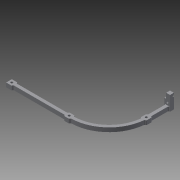
# Autodesk Inventor part: UndercarriageLeft
Saved by Autodesk Inventor 2014 SP1 (Build 180222100, 222)
## iProperties
Created: 2017-01-18
Part Number: UndercarriageLeft
Material: Generic
Document SubType Name: Modeling
Designer: danielsikar
Density: 1 g/cm^3
Appearance: Default
d38: 5.000 mm
d39: 200.000 mm
d40: 125.500 mm
d41: 11.000 mm
d42: 11.000 mm
d43: 11.000 mm
d44: 5.000 mm
d45: 6.000 mm
d46: 6.000 mm
d47: 150.000 mm
d48: 150.000 mm
d51: 6.000 mm
d52: 0.00 deg
d53: 4.300 mm
d54: 6.000 mm
d55: 0.00 deg
d56: 10.000 mm
d57: 0.00 deg
d58: 4.300 mm
d59: 5.000 mm
d60: 10.000 mm
d61: 0.00 deg
d62: 5.000 mm
d63: 10.000 mm
d64: 0.00 deg
d65: 4.300 mm
d66: 5.000 mm
d67: 10.000 mm
d68: 0.00 deg
d69: 11.000 mm
d70: 11.000 mm
d71: 6.000 mm
d72: 0.00 deg
d73: 4.300 mm
d74: 6.000 mm
d75: 0.00 deg
d76: 2.000 mm
d77: 2.000 mm
d80: 11.000 mm
d81: 11.000 mm
d82: 6.000 mm
d83: 0.00 deg
d84: 4.300 mm
d85: 6.000 mm
d86: 0.00 deg
d87: 2.000 mm
d88: 2.500 mm
d89: 0.00 deg
d98: 2.500 mm
d99: 0.00 deg
d100: 2.000 mm
d101: 2.000 mm
d102: 0.00 deg
Author: danielsikar
Autodesk Inventor part; units mm, degrees
ref_plane "YZ Plane" through (0, 0, 0) normal (1, 0, 0) x (0, 1, 0)
ref_plane "XZ Plane" through (0, 0, 0) normal (0, 1, 0) x (-1, 0, 0)
ref_plane "XY Plane" through (0, 0, 0) normal (0, 0, 1) x (1, 0, 0)
sketch "Sketch8" plane through (0, 0, 0) normal (0, 0, 1) x (1, 0, 0)
  line L0 (0, 0) -> (200, 0) construction
  line L1 (200, 0) -> (200, 125.5) construction
  line L2 (200, 125.5) -> (0, 125.5) construction
  line L3 (0, 125.5) -> (0, 0) construction
  line L4 (0, 0) -> (11, 0)
  line L5 (11, 11) -> (0, 11)
  line L6 (0, 11) -> (0, 0)
  line L7 (200, 125.5) -> (189, 125.5)
  line L8 (189, 125.5) -> (189, 120.5)
  line L9 (200, 120.5) -> (200, 125.5)
  line L10 (217.9822, 8.5) -> (217.9822, 2.5)
  line L11 (-10.7087, 2.5) -> (-10.7087, 8.5)
  line L12 (191.5, 137.3826) -> (197.5, 137.3826)
  line L13 (197.5, -11.2875) -> (191.5, -11.2875)
  line L14 (197.5, 2.5) -> (47.5, 2.5) construction
  line L15 (47.5, 2.5) -> (47.5, 152.5) construction
  line L16 (47.5, 152.5) -> (197.5, 152.5) construction
  line L17 (122.5, 152.5) -> (122.5, -14.6568) construction
  line L18 (47.5, 77.5) -> (239.0403, 77.5) construction
  circle A0 centre (122.5, 77.5) radius 69
  line L19 (-10.7087, 8.5) -> (0, 8.5)
  line L20 (217.9822, 2.5) -> (11, 2.5)
  line L21 (0, 2.5) -> (-10.7087, 2.5)
  line L22 (11, 0) -> (11, 2.5)
  line L23 (11, 8.5) -> (11, 11)
  line L24 (11, 8.5) -> (122.5, 8.5)
  line L25 (151.8939, 8.5) -> (217.9822, 8.5)
  line L26 (191.5, -11.2875) -> (191.5, 8.5)
  arc A1 (122.5, 2.5) -> (197.5, 77.5) centre (122.5, 77.5) ccw
  arc A2 (191.5, 106.8939) -> (93.1061, 8.5) centre (122.5, 77.5) ccw
  line L27 (189, 120.5) -> (191.5, 120.5)
  line L28 (197.5, 120.5) -> (200, 120.5)
  line L29 (191.5, 77.5) -> (191.5, 120.5)
  line L30 (191.5, 125.5) -> (191.5, 137.3826)
  line L31 (197.5, 152.5) -> (197.5, 125.5) construction
  line L32 (197.5, 120.5) -> (197.5, 2.5) construction
  line L33 (197.5, 137.3826) -> (197.5, 125.5)
  line L34 (197.5, 120.5) -> (197.5, 77.5)
  line L35 (197.5, 8.5) -> (197.5, -11.2875)
  point P0 (-10.7087, 5.5)
  point P1 (0, 5.5)
  point P2 (194.5, 137.3826)
  point P3 (194.5, 125.5)
  dimension "d39" = 200
  dimension "d40" = 125.5
  dimension "d41" = 11
  dimension "d42" = 11
  dimension "d43" = 11
  dimension "d44" = 5
  dimension "d45" = 6
  dimension "d46" = 6
  dimension "d47" = 150
  dimension "d48" = 150
  constraints: 72 end point, 28 parallel, 14 point on line, 13 perpendicular, 8 horizontal, 7 point on circle, 6 midpoint, 5 tangent, 3 centre point, 1 coincident, 1 horizontal alignment, 1 vertical alignment
  measures "d39" distance of L2.end L1.end
  measures "d40" distance of L1.end L0.end
  measures "d41" distance of L5.end L5.start
  measures "d42" distance of L5.start L4.end
  measures "d43" distance of L9.start L8.end
  measures "d44" distance of L8.end L7.end
  measures "d45" distance of L10.start L10.end
  measures "d46" distance of L13.start L13.end
  measures "d47" distance of L15.end L16.end
  measures "d48" distance of L14.end L15.end
extrude "Extrusion8" add sketch "Sketch8" along normal blind 6 contours L6 L5 L23 L24 A0 L29 L27 L8 L7 L9 L28 L34 A1 L20 L22 L4
sketch "Sketch9" plane through (0, 0, 6) normal (0, 0, 1) x (1, 0, 0)
  circle A0 centre (5.5, 5.5) radius 2.15
  dimension "d53" = 4.3
  constraints: 1 centre point
  measures "d53" diameter of A0
extrude "Extrusion9" cut sketch "Sketch9" against normal blind 6
sketch "Sketch10" plane through (0, 0, 6) normal (0, 0, 1) x (1, 0, 0)
  line L0 (189, 125.5) -> (200, 125.5)
  line L1 (200, 125.5) -> (200, 120.5)
  line L2 (200, 120.5) -> (189, 120.5)
  line L3 (189, 120.5) -> (189, 125.5)
  constraints: 8 end point, 2 parallel, 1 horizontal, 1 perpendicular
extrude "Extrusion10" add sketch "Sketch10" along normal blind 10
sketch "Sketch11" plane through (189, 125.5, 0) normal (0, 1, 0) x (1, 0, 0)
  line L0 (11, -16) -> (0, -16) projected
  circle A0 centre (5.5, -11) radius 2.15
  point P0 (-189, 0)
  dimension "d58" = 4.3
  dimension "d59" = 5
  constraints: 1 centre point
  measures "d58" diameter of A0
  measures "d59" distance from line of A0.centre L0
extrude "Extrusion11" cut sketch "Sketch11" against normal blind 10
sketch "Sketch12" plane through (0, 0, 16) normal (0, 0, 1) x (1, 0, 0)
  line L0 (189, 120.5) -> (200, 120.5) projected
  line L1 (200, 125.5) -> (195, 125.5)
  line L2 (195, 125.5) -> (195, 120.5)
  line L3 (195, 120.5) -> (200, 120.5)
  line L4 (200, 120.5) -> (200, 125.5)
  point P0 (0, 0)
  dimension "d62" = 5
  constraints: 8 end point, 2 parallel, 1 horizontal, 1 perpendicular, 1 point on line
  measures "d62" distance of L3.end L2.end
extrude "Extrusion12" add sketch "Sketch12" along normal blind 10
sketch "Sketch13" plane through (195, 120.5, 16) normal (-1, 0, 0) x (0, 0, 1)
  line L0 (10, 5) -> (10, 0) projected
  line L1 (0, 5) -> (10, 5) projected
  circle A0 centre (5, 5) radius 2.15
  point P0 (-16, -120.5)
  dimension "d65" = 4.3
  dimension "d66" = 5
  constraints: 1 centre point, 1 midpoint
  measures "d65" diameter of A0
  measures "d66" distance from line of L0 A0.centre
extrude "Extrusion13" cut sketch "Sketch13" against normal blind 10
sketch "Sketch14" plane through (0, 0, 6) normal (0, 0, 1) x (1, 0, 0)
  line L0 (0, 11) -> (0, 0) projected
  line L1 (122.5, 0) -> (111.5, 0)
  line L2 (111.5, 0) -> (111.5, 11)
  line L3 (111.5, 11) -> (122.5, 11)
  line L4 (122.5, 11) -> (122.5, 0)
  point P0 (111.5, 5.5)
  point P1 (0, 5.5)
  dimension "d69" = 11
  dimension "d70" = 11
  constraints: 8 end point, 2 midpoint, 2 parallel, 1 horizontal, 1 horizontal alignment, 1 perpendicular
  measures "d69" distance of L2.end L3.end
  measures "d70" distance between parallel lines of L1 L3
extrude "Extrusion14" add sketch "Sketch14" against normal blind 6
sketch "Sketch15" plane through (0, 0, 6) normal (0, 0, 1) x (1, 0, 0)
  circle A0 centre (117, 5.5) radius 2.15
  dimension "d73" = 4.3
  constraints: 1 centre point
  measures "d73" diameter of A0
extrude "Extrusion15" cut sketch "Sketch15" against normal blind 6
fillet "Fillet1" radius 2 7 edges at (122.5, 0, 3) (122.5, 2.5, 3) (122.5, 11, 3) (122.5, 8.5, 3) (111.5, 0, 3) (111.5, 8.5, 3) (111.5, 11, 3)
fillet "Fillet2" radius 2 2 edges at (11, 2.5, 3) (11, 8.5, 3)
sketch "Sketch16" plane through (0, 0, 6) normal (0, 0, 1) x (1, 0, 0)
  arc A0 (124.4481, 2.5253) -> (197.5, 77.5) centre (122.5, 77.5) ccw projected
  line L0 (197.5, 120.5) -> (191.5, 120.5) projected
  line L1 (189, 83) -> (200, 83)
  line L2 (200, 83) -> (200, 72)
  line L3 (200, 72) -> (189, 72)
  line L4 (189, 72) -> (189, 83)
  point P0 (199.5, 120.5)
  point P1 (189.5, 120.5)
  point P2 (189, 77.5)
  point P3 (194.5, 83)
  point P4 (194.5, 120.5)
  dimension "d80" = 11
  dimension "d81" = 11
  constraints: 8 end point, 3 midpoint, 2 parallel, 1 horizontal, 1 horizontal alignment, 1 perpendicular, 1 vertical alignment
  measures "d80" distance of L2.end L3.end
  measures "d81" distance of L1.end L2.end
extrude "Extrusion16" add sketch "Sketch16" against normal blind 6
sketch "Sketch17" plane through (0, 0, 6) normal (0, 0, 1) x (1, 0, 0)
  circle A0 centre (194.5, 77.5) radius 2.15
  dimension "d84" = 4.3
  constraints: 1 centre point
  measures "d84" diameter of A0
extrude "Extrusion17" cut sketch "Sketch17" against normal blind 6
fillet "Fillet5" radius 2 8 edges at (197.5, 83, 3) (200, 83, 3) (191.5, 83, 3) (189, 83, 3) (189, 72, 3) (191.2804, 72, 3) (200, 72, 3) (197.2981, 72, 3)
sketch "Sketch18" plane through (189, 120.5, 0) normal (0, -1, 0) x (1, 0, 0)
  circle A0 centre (5.5, 11) radius 2.15 projected
  line L0 (0, 0) -> (2.5, 0) projected
  line L1 (2.5, 0) -> (2.5, 6) projected
  line L2 (8.5, 6) -> (2.5, 6) projected
  line L3 (8.5, 0) -> (8.5, 6) projected
  line L4 (8.5, 0) -> (11, 0) projected
  line L5 (11, 0) -> (11, 26) projected
  line L6 (6, 26) -> (11, 26) projected
  line L7 (6, 16) -> (6, 26) projected
  line L8 (0, 16) -> (6, 16) projected
  line L9 (0, 0) -> (0, 16) projected
  point P0 (-189, 0)
extrude "Extrusion18" add sketch "Sketch18" along normal blind 2.5
sketch "Sketch22" plane through (195, 125.5, 21) normal (-1, 0, 0) x (0, 0, 1)
  arc A0 (-2.15, 0) -> (2.15, 0) centre (0, 0) ccw projected
  line L0 (-5, 0) -> (-2.15, 0) projected
  line L1 (-5, -7.5) -> (-5, 0) projected
  line L2 (5, -7.5) -> (-5, -7.5) projected
  line L3 (5, 0) -> (5, -7.5) projected
  line L4 (2.15, 0) -> (5, 0) projected
  point P0 (-21, -125.5)
extrude "Extrusion22" add sketch "Sketch22" along normal blind 2.5
fillet "Fillet8" radius 2 2 edges at (191.5, 118, 3) (197.5, 118, 3)
sketch "Sketch23" plane through (0, 0, 0) normal (0, 0, -1) x (-1, 0, 0)
  circle A0 centre (-5.5, 5.5) radius 2.15 projected
  circle A1 centre (-117, 5.5) radius 2.15 projected
  circle A2 centre (-194.5, 77.5) radius 2.15 projected
  arc A3 (-200, 73.8359) -> (-198.5669, 71.918) centre (-198, 73.8359) ccw projected
  arc A4 (-197.1434, 70.1948) -> (-198.5669, 71.918) centre (-199.1339, 70) ccw projected
  arc A5 (-197.1434, 70.1948) -> (-124.4481, 2.5253) centre (-122.5, 77.5) ccw projected
  arc A6 (-122.6407, 1.263) -> (-124.4481, 2.5253) centre (-124.5, 0.526) ccw projected
  arc A7 (-122.6407, 1.263) -> (-120.7815, 0) centre (-120.7815, 2) ccw projected
  line L0 (-120.7815, 0) -> (-113.5, 0) projected
  arc A8 (-113.5, 0) -> (-111.5, 2) centre (-113.5, 2) ccw projected
  line L1 (-111.5, 2) -> (-111.5, 2.5) projected
  line L2 (-13, 2.5) -> (-111.5, 2.5) projected
  arc A9 (-11, 0.5) -> (-13, 2.5) centre (-13, 0.5) ccw projected
  line L3 (-11, 0) -> (-11, 0.5) projected
  line L4 (0, 0) -> (-11, 0) projected
  line L5 (0, 11) -> (0, 0) projected
  line L6 (-11, 11) -> (0, 11) projected
  line L7 (-11, 10.5) -> (-11, 11) projected
  arc A10 (-13, 8.5) -> (-11, 10.5) centre (-13, 10.5) ccw projected
  line L8 (-109.5, 8.5) -> (-13, 8.5) projected
  arc A11 (-111.354, 9.75) -> (-109.5, 8.5) centre (-109.5, 10.5) ccw projected
  arc A12 (-111.354, 9.75) -> (-113.2081, 11) centre (-113.2081, 9) ccw projected
  line L9 (-113.2081, 11) -> (-120.5, 11) projected
  arc A13 (-120.5, 11) -> (-122.3497, 9.7608) centre (-120.5, 9) ccw projected
  arc A14 (-124.25, 8.5222) -> (-122.3497, 9.7608) centre (-124.1993, 10.5216) ccw projected
  arc A15 (-191.0663, 69.7761) -> (-124.25, 8.5222) centre (-122.5, 77.5) ccw projected
  arc A16 (-190.0395, 71.7542) -> (-191.0663, 69.7761) centre (-189.0789, 70) ccw projected
  arc A17 (-190.0395, 71.7542) -> (-189, 73.5085) centre (-191, 73.5085) ccw projected
  line L10 (-189, 73.5085) -> (-189, 81.2919) projected
  arc A18 (-189, 81.2919) -> (-190.25, 83.146) centre (-191, 81.2919) ccw projected
  arc A19 (-191.5, 85) -> (-190.25, 83.146) centre (-189.5, 85) ccw projected
  line L11 (-191.5, 116) -> (-191.5, 85) projected
  arc A20 (-189.5, 118) -> (-191.5, 116) centre (-189.5, 116) ccw projected
  line L12 (-189, 118) -> (-189.5, 118) projected
  line L13 (-189, 125.5) -> (-189, 118) projected
  line L14 (-200, 125.5) -> (-189, 125.5) projected
  line L15 (-200, 125.5) -> (-200, 118) projected
  line L16 (-199.5, 118) -> (-200, 118) projected
  arc A21 (-197.5, 116) -> (-199.5, 118) centre (-199.5, 116) ccw projected
  line L17 (-197.5, 85) -> (-197.5, 116) projected
  arc A22 (-198.75, 83.146) -> (-197.5, 85) centre (-199.5, 85) ccw projected
  arc A23 (-198.75, 83.146) -> (-200, 81.2919) centre (-198, 81.2919) ccw projected
  line L18 (-200, 81.2919) -> (-200, 73.8359) projected
extrude "Extrusion23" add sketch "Sketch23" along normal blind 2
body "Solid4"
